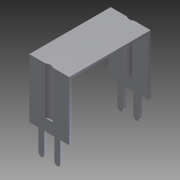
# Autodesk Inventor part: BBRACKET13
Saved by Autodesk Inventor 2011 SP1 (Build 150282100, 282)
## iProperties
Created: 2013-12-24
Part Number: BBRACKET13
Catalog Web Link: www.cadenas.de
Description: M BR BRACKET BRACKET-Series M
Vendor: NKKSWITCHES
Document SubType Name: Modeling
Designer: PARTuser1
Manufacturer: NKKSWITCHES
Density: 1 g/cm^3
Category: PARTsolutions
Company: NKKSWITCHES
Title: BBRACKET13
Author: Cadenas PARTsolutions
Comments: Series M
PSOL_IDENT_0: {$CADENAS_DATA\23d-libs\nkkswitches\toggle\m\parts\m_br_bracket.prj},182 {VTYP=3D},{NB=BBRACKET13},{
PSOL_IDENT_1: LINA=BBRACKET13},{NN=M BR BRACKET BRACKET},{DATE=10.11.2009 13:43:08},{GEOMDATE=10.11.2009 00:00:00}
PSOL_IDENT_2: ,{VERSION=},{LINEID=10},{LINESUBID=-1},{WBVAR=TRMNLS}  {NB=BBRACKET13},{LINA=BBRACKET13},{KT=DUMMY},
PSOL_IDENT_3: {PN=BBRACKET13},{A=0.62200},{B=0.02000},{C=0.31500},{BR=B},{TRMNLS=13},{TRMNLALG='13','13 - .250\" (
PSOL_IDENT_4: 6.35mm) Straight PC with .465\" (11.8mm) Bracket','15','15 - .425\" (10.8mm) Straight PC with .630\"
PSOL_IDENT_5: (16.0mm) Bracket','17','17 - .964\" (24.5mm) Straight PC with 1.150\" (29.2mm) Bracket'},{HEIGHT=0.
PSOL_IDENT_6: 465},{E=0.12600}
CNS_NN: M BR BRACKET BRACKET
CNS_NT: Series M
CNS_NB: BBRACKET13
CNS_NBSYN: $PN.
CNS_LINA: BBRACKET13
CNS_PN: BBRACKET13
CNS_A: 0.62200
CNS_B: 0.02000
CNS_C: 0.31500
CNS_BR: B
CNS_TRMNLS: 13 - .250" (6.35mm) Straight PC with .465" (11.8mm) Bracket
CNS_TRMNLALG: '13','13 - .250" (6.35mm) Straight PC with .465" (11.8mm) Bracket','15','15 - .425" (10.8mm) Straight PC with .630" (16.0mm) Bracket','17','17 - .964" (24.5mm) Straight PC with 1.150" (29.2mm) Bracket'
CNS_HEIGHT: 0.465
CNS_E: 0.12600
SUPPLIER: NKKSWITCHES
ARTICLENO: BBRACKET13
BOMINFO: BBRACKET13
CREATOR: CADENAS GmbH
Autodesk Inventor part; units mm, degrees
sketch "Sketch_1" plane through (0, 0, 0) normal (1, 0, 0) x (0, 1, 0)
  line L0 (-4.8006, 8.1534) -> (-4.8006, 7.6454)
  line L1 (-4.8006, 7.6454) -> (11.303, 7.6454)
  line L2 (11.303, 7.6454) -> (11.303, -7.6454)
  line L3 (11.303, -7.6454) -> (-4.8006, -7.6454)
  line L4 (-4.8006, -7.6454) -> (-4.8006, -8.1534)
  line L5 (-4.8006, -8.1534) -> (11.811, -8.1534)
  line L6 (11.811, -8.1534) -> (11.811, 8.1534)
  line L7 (11.811, 8.1534) -> (-4.8006, 8.1534)
  constraints: 16 end point
extrude "Extrusion1" add sketch "Sketch_1" along normal mid plane 8.001
sketch "Sketch_2" plane through (0, 0, 0) normal (0, 0, 1) x (1, 0, 0)
  line L0 (-4.0005, 0) -> (-4.0005, -4.953)
  line L1 (-4.0005, -4.953) -> (4.0005, -4.953)
  line L2 (4.0005, -4.953) -> (4.0005, 0)
  line L3 (4.0005, 0) -> (2.1844, 0)
  line L4 (2.1844, 0) -> (2.1844, -4.2164)
  arc A0 (1.016, -4.2164) -> (2.1844, -4.2164) centre (1.6002, -4.2164) ccw
  line L5 (1.016, -4.2164) -> (1.016, 0)
  line L6 (1.016, 0) -> (-1.016, 0)
  line L7 (-1.016, 0) -> (-1.016, -4.2164)
  arc A1 (-2.1844, -4.2164) -> (-1.016, -4.2164) centre (-1.6002, -4.2164) ccw
  line L8 (-2.1844, -4.2164) -> (-2.1844, 0)
  line L9 (-2.1844, 0) -> (-4.0005, 0)
  constraints: 20 end point, 4 point on circle, 2 centre point
extrude "Extrusion2" cut sketch "Sketch_2" along normal mid plane 16.3068
sketch "Sketch_3" plane through (0, 2.3622, 0) normal (0, 1, 0) x (1, 0, 0)
  arc A0 (-0.762, 7.6454) -> (0.762, 7.6454) centre (0, 8.6614) ccw
  line L0 (0.762, 7.6454) -> (-0.762, 7.6454)
  constraints: 2 end point, 2 point on circle, 1 centre point
extrude "Extrusion3" add sketch "Sketch_3" along normal blind 9.4488
sketch "Sketch_4" plane through (0, 2.3622, 0) normal (0, 1, 0) x (1, 0, 0)
  arc A0 (-1.27, 9.1694) -> (1.27, 9.1694) centre (0, 9.1694) ccw
  line L0 (1.27, 9.1694) -> (-1.27, 9.1694)
  constraints: 2 end point, 2 point on circle, 1 centre point
extrude "Extrusion4" cut sketch "Sketch_4" along normal blind 9.4488
sketch "Sketch_5" plane through (0, 2.3622, 0) normal (0, 1, 0) x (1, 0, 0)
  line L0 (-0.907, -7.6454) -> (0.907, -7.6454)
  arc A0 (0.907, -7.6454) -> (-0.907, -7.6454) centre (0, -8.5344) ccw
  constraints: 2 end point, 2 point on circle, 1 centre point
extrude "Extrusion5" add sketch "Sketch_5" along normal blind 9.4488
sketch "Sketch_6" plane through (0, 2.3622, 0) normal (0, 1, 0) x (1, 0, 0)
  line L0 (-1.27, -9.1694) -> (1.27, -9.1694)
  arc A0 (1.27, -9.1694) -> (-1.27, -9.1694) centre (0, -9.1694) ccw
  constraints: 2 end point, 2 point on circle, 1 centre point
extrude "Extrusion6" cut sketch "Sketch_6" along normal blind 9.4488
ref_plane "bracket_to_switch_XY" through (0, 11.303, 0) normal (0, 1, 0) x (1, 0, 0)
ref_plane "bracket_to_switch_YZ" through (0, 11.303, 0) normal (1, 0, 0) x (0, 0, -1)
ref_plane "bracket_to_switch_ZX" through (0, 11.303, 0) normal (0, 0, -1) x (0, 1, 0)
body "Solid1"
